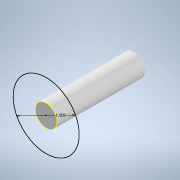
# Autodesk Inventor part: innerClutch
Saved by Autodesk Inventor 2021 (Build 250183000, 183)
## iProperties
Created: 2020-06-28
Part Number: innerClutch
Material: PET Plastic
Document SubType Name: Modeling
Designer: robst
Density: 1.541 g/cm^3
Appearance: Smooth - Yellow
Author: robst
Autodesk Inventor part; units mm, degrees
ref_plane "YZ Plane" through (0, 0, 0) normal (1, 0, 0) x (0, 1, 0)
ref_plane "XZ Plane" through (0, 0, 0) normal (0, 1, 0) x (-1, 0, 0)
ref_plane "XY Plane" through (0, 0, 0) normal (0, 0, 1) x (1, 0, 0)
sketch "Sketch1" plane through (0, 0, 0) normal (0, 0, 1) x (1, 0, 0)
  circle A0 centre (0, 0) radius 6.35
  dimension "d0" = 12.7
  constraints: 1 centre point, 1 coincident
  measures "d0" diameter of A0
extrude "Extrusion1" add sketch "Sketch1" against normal blind 50.8
sketch "Sketch2" plane through (0, 0, 0) normal (0, 0, 1) x (1, 0, 0)
  circle A0 centre (0, 0) radius 6.35 projected
  circle A1 centre (0, 0) radius 19.05
  dimension "d3" = 38.1
  constraints: 1 centre point, 1 coincident
  measures "d3" diameter of A1
extrude "Extrusion2" add sketch "Sketch2" against normal blind 6.35
sketch "Sketch4" plane through (0, 0, -6.35) normal (0, 0, -1) x (-1, 0, 0)
  circle A0 centre (0, 0) radius 19.05 projected
  circle A1 centre (0, 0) radius 6.35 construction
  line L0 (0, 0) -> (0, 19.05) construction
  circle A2 centre (0, 0) radius 19.05 construction
  line L1 (-3.175, 18.7836) -> (-3.175, 15.6086)
  line L2 (-3.175, 15.6086) -> (0, 15.6086)
  line L3 (3.175, 18.7836) -> (3.175, 15.6086)
  line L4 (3.175, 15.6086) -> (0, 15.6086)
  arc A3 (3.175, 18.7836) -> (-3.175, 18.7836) centre (0, 0) ccw
  dimension "d6" = 3.175
  dimension "d7" = 3.175
  constraints: 10 end point, 4 point on circle, 2 symmetric about line, 2 vertical, 1 centre point, 1 coincident, 1 concentric, 1 perpendicular, 1 point on line
  measures "d6" distance of L1.start L1.end
  measures "d7" distance of L1.end L2.end
extrude "Extrusion3" add sketch "Sketch4" along normal blind 25.4 contours L3 L4 L2 L1 A0 picked at (-1.4126, 16.7458)
body "Solid1"
